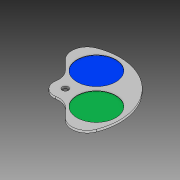
# Autodesk Inventor part: FILTER WHEEL
Saved by Autodesk Inventor 2017 (Build 210142000, 142)
## iProperties
Created: 2017-04-01
Part Number: FILTER WHEEL
Material: Generic
Document SubType Name: Modeling
Designer: Muchen
Density: 1 g/cm^3
Appearance: Default
Author: Muchen
Autodesk Inventor part; units mm, degrees
ref_plane "YZ Plane" through (0, 0, 0) normal (1, 0, 0) x (0, 1, 0)
ref_plane "XZ Plane" through (0, 0, 0) normal (0, 1, 0) x (-1, 0, 0)
ref_plane "XY Plane" through (0, 0, 0) normal (0, 0, 1) x (1, 0, 0)
sketch "Sketch1" plane through (0, 0, 0) normal (0, 0, 1) x (1, 0, 0)
  circle A0 centre (0, 0) radius 40 construction
  circle A1 centre (0, 40) radius 25
  circle A2 centre (40, 0) radius 25
  circle A3 centre (0, 0) radius 70
  line L0 (-49.4975, 49.4975) -> (-10.6066, 10.6066)
  line L1 (40, 0) -> (0, 0) construction
  arc A4 (2.8284, -2.8284) -> (-2.8284, 2.8284) centre (0, 0) ccw
  circle A5 centre (0, 0) radius 15
  line L2 (-10.6066, 10.6066) -> (10.6066, -10.6066)
  line L3 (10.6066, -10.6066) -> (49.4975, -49.4975)
  arc A6 (-2.8284, 2.8284) -> (2.8284, -2.8284) centre (0, 0) ccw
  dimension "d0" = 50
  dimension "d1" = 50
  dimension "d2" = 30
  dimension "d3" = 45
  dimension "d4" = 80
  dimension "d5" = 8
  dimension "d6" = 30
  constraints: 10 point on circle, 8 end point, 7 centre point, 3 coincident, 3 point on line, 1 collinear, 1 horizontal, 1 horizontal alignment, 1 midpoint, 1 vertical alignment
  measures "d0" diameter of A1
  measures "d1" diameter of A2
  measures "d2" radial gap between concentric circles of A0 A3
  measures "d3" angle of L0 L1
  measures "d4" diameter of A0
  measures "d5" diameter of A4
  measures "d6" diameter of A5
extrude "Extrusion1" add sketch "Sketch1" along normal mid plane 3 contours A5 L0 A3 L3 | A5 L2 A4 | L2 A6 A5 picked at (36.2103, 39.0042)
fillet "Fillet1" radius 20 8 edges at (-49.4975, 49.4975, 0.75) (-49.4975, 49.4975, -0.75) (49.4975, -49.4975, 0.75) (49.4975, -49.4975, -0.75) (10.6066, -10.6066, 0.75) (10.6066, -10.6066, -0.75) (-10.6066, 10.6066, 0.75) (-10.6066, 10.6066, -0.75)
sketch "Sketch2" plane through (0, 0, 0) normal (1, 0, 0) x (0, 1, 0)
  line L0 (40, 10.9334) -> (40, -11.9081)
  line L1 (65, -1.5) -> (15, -1.5) construction
  line L2 (15, 1.5) -> (65, 1.5) construction
  line L3 (65, -1.5) -> (65, 1.5) construction
  line L4 (65, 1) -> (65, -1)
  arc A0 (65, 1) -> (40, 1.5) centre (40, -623.75) ccw
  arc A1 (40, -1.5) -> (65, -1) centre (40, 623.75) ccw
  line L5 (40, 1.5) -> (40, -1.5)
  point P0 (0, 0)
  point P1 (65, 0)
  point P2 (65, 0)
  dimension "d10" = 2
  constraints: 6 end point, 4 midpoint, 4 point on circle, 2 centre point, 2 line through centre, 2 point on line, 1 coincident, 1 collinear, 1 vertical, 1 vertical alignment
  measures "d10" distance of L4.end L4.start
revolve "Revolution1" add sketch "Sketch2" angle 360 about axis through (0, 40, 10.9334) along (0, 0, -1)
pattern_circular "Circular Pattern1" count 2 over 90 about axis through (0, 0, -10) along (0, 0, -1) of "Revolution1"
body "Solid1"
